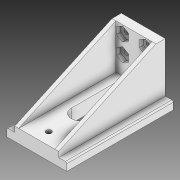
# Autodesk Inventor part: 1322_Clamp Holder_V1
Saved by Autodesk Inventor 2020 (Build 240168000, 168)
## iProperties
Created: 2019-10-02
Part Number: 1322_Clamp Holder_V1
Material: Acetal Resin, White
Document SubType Name: Modeling
Designer: MPI
Density: 1.425 g/cm^3
Appearance: Smooth - White
Author: MPI
Autodesk Inventor part; units mm, degrees
ref_plane "YZ Plane" through (0, 0, 0) normal (1, 0, 0) x (0, 1, 0)
ref_plane "XZ Plane" through (0, 0, 0) normal (0, 1, 0) x (-1, 0, 0)
ref_plane "XY Plane" through (0, 0, 0) normal (0, 0, 1) x (1, 0, 0)
sketch "Sketch1" plane through (0, 0, 0) normal (0, 0, 1) x (1, 0, 0)
  line L0 (0, 43.4) -> (27, 43.4)
  line L1 (27, 43.4) -> (27, 0)
  line L2 (27, 0) -> (0, 0)
  line L3 (0, 0) -> (0, 43.4)
  circle A0 centre (5, 37.4) radius 2
  circle A1 centre (22, 37.4) radius 2
  circle A2 centre (5, 23.91) radius 2
  circle A3 centre (22, 23.91) radius 2
  dimension "d0" = 27
  dimension "d1" = 43.4
  dimension "d2" = 4
  dimension "d3" = 6
  dimension "d4" = 6
  dimension "d5" = 5
  dimension "d6" = 5
  dimension "d7" = 5
  dimension "d8" = 5
  dimension "d61" = 13.49
  dimension "d62" = 13.49
  constraints: 8 end point, 4 centre point, 3 equal radius, 2 parallel, 1 coincident, 1 horizontal, 1 perpendicular
  measures "d0" distance of L0.start L0.end
  measures "d1" distance of L2.end L0.start
  measures "d2" diameter of A0
  measures "d3" distance from line of L0 A0.centre
  measures "d4" distance from line of A1.centre L0
  measures "d5" distance from line of L3 A0.centre
  measures "d6" distance from line of A1.centre L1
  measures "d7" distance from line of L1 A3.centre
  measures "d8" distance from line of L3 A2.centre
  measures "d61" distance of A2.centre A0.centre
  measures "d62" distance of A3.centre A1.centre
extrude "Extrusion1" add sketch "Sketch1" along normal blind 7
sketch "Sketch2" plane through (0, 0, 7) normal (0, 0, 1) x (1, 0, 0)
  line L0 (0, 10) -> (27, 10)
  line L1 (27, 10) -> (27, 0)
  line L2 (27, 0) -> (0, 0)
  line L3 (0, 0) -> (0, 10)
  line L4 (0, 0) -> (27, 0) projected
  line L5 (0, 43.4) -> (0, 0) projected
  line L6 (27, 0) -> (27, 43.4) projected
  dimension "d13" = 10
  constraints: 8 end point, 3 collinear, 2 parallel, 1 horizontal, 1 perpendicular
  measures "d13" distance of L2.end L0.start
extrude "Extrusion2" add sketch "Sketch2" along normal blind 73
sketch "Sketch3" plane through (0, 0, 7) normal (0, 0, 1) x (1, 0, 0)
  line L0 (0.5, 39.9981) -> (0.5, 34.8019)
  line L1 (0.5, 34.8019) -> (5, 32.2038)
  line L2 (5, 32.2038) -> (9.5, 34.8019)
  line L3 (9.5, 34.8019) -> (9.5, 39.9981)
  line L4 (9.5, 39.9981) -> (5, 42.5962)
  line L5 (5, 42.5962) -> (0.5, 39.9981)
  circle A0 centre (5, 37.4) radius 4.5
  circle A1 centre (5, 37.4) radius 2 projected
  line L6 (17.5, 39.9981) -> (17.5, 34.8019)
  line L7 (17.5, 34.8019) -> (22, 32.2038)
  line L8 (22, 32.2038) -> (26.5, 34.8019)
  line L9 (26.5, 34.8019) -> (26.5, 39.9981)
  line L10 (26.5, 39.9981) -> (22, 42.5962)
  line L11 (22, 42.5962) -> (17.5, 39.9981)
  circle A2 centre (22, 37.4) radius 4.5
  line L12 (17.5, 26.5081) -> (17.5, 21.3119)
  line L13 (17.5, 21.3119) -> (22, 18.7138)
  line L14 (22, 18.7138) -> (26.5, 21.3119)
  line L15 (26.5, 21.3119) -> (26.5, 26.5081)
  line L16 (26.5, 26.5081) -> (22, 29.1062)
  line L17 (22, 29.1062) -> (17.5, 26.5081)
  circle A3 centre (22, 23.91) radius 4.5
  line L18 (0.5, 26.5081) -> (0.5, 21.3119)
  line L19 (0.5, 21.3119) -> (5, 18.7138)
  line L20 (5, 18.7138) -> (9.5, 21.3119)
  line L21 (9.5, 21.3119) -> (9.5, 26.5081)
  line L22 (9.5, 26.5081) -> (5, 29.1062)
  line L23 (5, 29.1062) -> (0.5, 26.5081)
  circle A4 centre (5, 23.91) radius 4.5
  circle A5 centre (22, 37.4) radius 2 projected
  circle A6 centre (22, 23.91) radius 2 projected
  circle A7 centre (5, 23.91) radius 2 projected
  point P0 (0, 0)
  dimension "d16" = 120
  dimension "d17" = 120
  dimension "d18" = 9
  dimension "d19" = 120
  dimension "d20" = 120
  dimension "d21" = 9
  dimension "d22" = 120
  dimension "d23" = 120
  dimension "d24" = 9
  dimension "d25" = 120
  dimension "d26" = 120
  dimension "d27" = 9
  constraints: 48 end point, 16 equal length, 12 tangent, 8 parallel, 4 centre point, 4 concentric, 4 vertical
  measures "d16" angle of L5 L4
  measures "d17" angle of L0 L5
  measures "d18" distance between parallel lines of L3 L0
  measures "d19" angle of L11 L10
  measures "d20" angle of L6 L11
  measures "d21" distance between parallel lines of L9 L6
  measures "d22" angle of L17 L16
  measures "d23" angle of L12 L17
  measures "d24" distance between parallel lines of L15 L12
  measures "d25" angle of L23 L22
  measures "d26" angle of L18 L23
  measures "d27" distance between parallel lines of L21 L18
extrude "Extrusion3" cut sketch "Sketch3" against normal blind 3 contours L5 A0 L0 | A0 L1 L0 | A0 | L5 L4 A0 | A0 L2 L1 | L4 L3 A0 | A0 L3 L2 | A1 | L11 A2 L6 | A2 L7 L6 | A2 | L11 L10 A2 | A2 L8 L7 | L10 L9 A2 | A2 L9 L8 | L17 A3 L12 | A3 L13 L12 | A3 | L17 L16 A3 | A3 L14 L13 | L16 L15 A3 | A3 L15 L14 | L23 A4 L18 | A4 L19 L18 | A4 | L23 L22 A4 | A4 L20 L19 | L22 L21 A4 | A4 L21 L20 | A5 | A6 | A7
sketch "Sketch4" plane through (27, 0, 0) normal (1, 0, 0) x (0, 0, -1)
  line L0 (-80, 10) -> (-80, 0) projected
  line L1 (-7, 43.4) -> (-80, 10)
  line L2 (-80, 10) -> (-80, 0)
  line L3 (0, 43.4) -> (0, 0) projected
  line L4 (-80, 0) -> (0, 0)
  line L5 (0, 0) -> (0, 43.4)
  line L6 (0, 43.4) -> (-7, 43.4) projected
  line L7 (0, 43.4) -> (-7, 43.4)
  constraints: 10 end point, 2 collinear, 2 perpendicular
extrude "Extrusion4" add sketch "Sketch4" along normal blind 3
sketch "Sketch5" plane through (0, 0, 0) normal (-1, 0, 0) x (0, 0, 1)
  line L0 (80, 0) -> (0, 0) projected
  line L1 (80, 10) -> (80, 0) projected
  line L2 (80, 0) -> (80, 10)
  line L3 (7, 43.4) -> (80, 10) projected
  line L4 (80, 10) -> (7, 43.4)
  line L5 (0, 43.4) -> (7, 43.4) projected
  line L6 (7, 43.4) -> (0, 43.4)
  line L7 (0, 43.4) -> (0, 0) projected
  line L8 (0, 43.4) -> (0, 0)
  line L9 (0, 0) -> (80, 0)
  constraints: 10 end point, 4 collinear, 1 perpendicular
extrude "Extrusion5" add sketch "Sketch5" along normal blind 3
sketch "Sketch6" plane through (27, 10, 80) normal (0, 1, 0) x (1, 0, 0)
  circle A0 centre (-13.5, 9) radius 2
  line L0 (-27, 0) -> (-27, 73) projected
  line L1 (0, 0) -> (-27, 0) projected
  line L2 (-30, 80) -> (3, 80) projected
  point P0 (-27, 80)
  dimension "d34" = 4
  dimension "d35" = 13.5
  dimension "d45" = 71
  constraints: 1 centre point
  measures "d34" diameter of A0
  measures "d35" distance from line of L0 A0.centre
  measures "d45" distance from line of A0.centre L2
extrude "Extrusion6" cut sketch "Sketch6" against normal blind 74
sketch "Sketch7" plane through (30, 0, 0) normal (0, -1, 0) x (1, 0, 0)
  line L0 (-9.5, 47) -> (-9.5, 0)
  line L1 (-9.5, 0) -> (-23.5, 0)
  line L2 (-23.5, 0) -> (-23.5, 47)
  line L3 (0, 80) -> (0, 0) projected
  line L4 (-33, 0) -> (-33, 80) projected
  line L5 (-33, 0) -> (0, 0) projected
  arc A0 (-9.5, 47) -> (-23.5, 47) centre (-16.5, 47) ccw
  point P0 (-30, 0)
  dimension "d39" = 33
  dimension "d40" = 14
  dimension "d41" = 9.5
  dimension "d42" = 47
  constraints: 6 end point, 2 point on circle, 1 centre point, 1 collinear, 1 parallel
  measures "d39" distance between parallel lines of L3 L4
  measures "d40" distance of L2.end L0.start
  measures "d41" distance between parallel lines of L2 L4
  measures "d42" distance of L0.start L0.end
extrude "Extrusion7" cut sketch "Sketch7" against normal blind 10
sketch "Sketch8" plane through (0, 0, 0) normal (0, 0, -1) x (-1, 0, 0)
  line L0 (-27, 10) -> (0, 10) projected
  circle A0 centre (-13.5, 10) radius 7
  point P0 (0, 0)
  point P1 (-6.5, 10)
  point P2 (-20.5, 10)
  constraints: 2 point on circle, 1 centre point, 1 midpoint
extrude "Extrusion8" cut sketch "Sketch8" against normal blind 74 contours A0 L0 picked at (-15.8333, 12.1687)
sketch "Sketch10" plane through (0, 0, 0) normal (0, 0, -1) x (-1, 0, 0)
  line L0 (3, 6) -> (9, 6)
  line L1 (9, 6) -> (9, 0)
  line L2 (9, 0) -> (3, 0)
  line L3 (3, 0) -> (3, 6)
  line L4 (3, 0) -> (-6.5, 0) projected
  line L5 (3, 43.4) -> (3, 0) projected
  line L6 (-36, 6) -> (-30, 6)
  line L7 (-30, 6) -> (-30, 0)
  line L8 (-30, 0) -> (-36, 0)
  line L9 (-36, 0) -> (-36, 6)
  point P0 (0, 0)
  point P1 (-30, 0)
  dimension "d56" = 6
  dimension "d57" = 6
  constraints: 16 end point, 4 collinear, 4 parallel, 2 horizontal, 2 perpendicular, 1 coincident
  measures "d56" distance of L0.end L1.end
  measures "d57" distance of L0.start L0.end
extrude "Extrusion10" add sketch "Sketch10" against normal up to surface (80 mm away)
fillet "Fillet1" radius 1 2 edges at (-9, 6, 40) (36, 6, 40)
body "Solid1"
